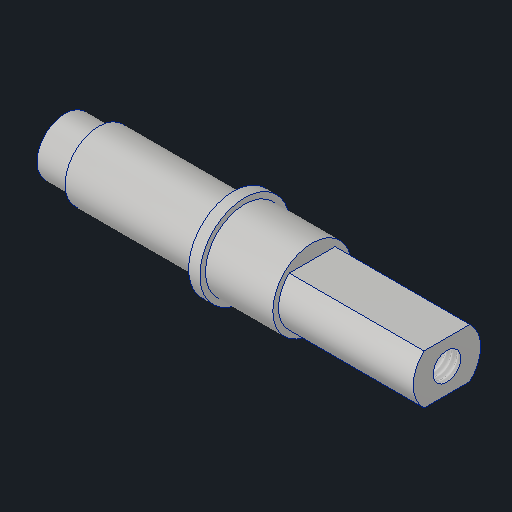
# Autodesk Inventor part: Wał koła
Saved by Autodesk Inventor 2023 (Build 270158000, 158)
## iProperties
Created: 2020-02-09
Part Number: Wał koła
Material: Aluminum 6061
Document SubType Name: Modeling
Designer: SKYNET
Density: 2.7 g/cm^3
Appearance: Aluminum - Flat
Mass: 2.47378 g
Surface Area: 8.25416 cm^2
Volume: 0.916215 cm^3
Author: SKYNET
Autodesk Inventor part; units mm, degrees
ref_plane "YZ Plane" through (0, 0, 0) normal (1, 0, 0) x (0, 1, 0)
ref_plane "XZ Plane" through (0, 0, 0) normal (0, 1, 0) x (-1, 0, 0)
ref_plane "XY Plane" through (0, 0, 0) normal (0, 0, 1) x (1, 0, 0)
sketch "Sketch1" plane through (0, 0, 0) normal (0, 0, 1) x (1, 0, 0)
  line L0 (4, 3) -> (6, 3)
  line L1 (6, 3) -> (6, 3)
  line L2 (16.5, 3.5) -> (16.5, 3.5)
  line L3 (35, 3) -> (35, 0)
  line L4 (4, 3) -> (4, 2.5)
  line L5 (4, 2.5) -> (1, 2.5)
  line L6 (1, 2.5) -> (1, 0)
  line L7 (1, 0) -> (35, 0)
  line L8 (23, 3) -> (35, 3)
  line L9 (23, 3.5) -> (17, 3.5)
  line L10 (23, 3.5) -> (23, 3)
  line L11 (17, 3.5) -> (17, 4)
  line L12 (17, 4) -> (16, 4)
  line L13 (16, 4) -> (16, 3)
  line L14 (6, 3) -> (16, 3)
  point P0 (0, 0)
  dimension "d1" = 2
  dimension "d25" = 3
  dimension "d26" = 2.5
  dimension "d40" = 12
  dimension "d41" = 3
  dimension "d42" = 0.5
  dimension "d44" = 6
  dimension "d45" = 1
  dimension "d46" = 10
  dimension "d47" = 3
  dimension "d48" = 3
  constraints: 30 end point, 6 horizontal, 6 vertical, 4 perpendicular
  measures "d1" distance of L0.start L0.end
  measures "d25" distance of L4.end L5.end
  measures "d26" distance of L5.end L6.end
  measures "d40" distance of L8.start L3.start
  measures "d41" distance of L3.start L3.end
  measures "d42" distance of L9.end L11.end
  measures "d44" distance of L9.start L9.end
  measures "d45" distance of L11.end L12.end
  measures "d46" distance of L1.end L13.end
  measures "d47" distance between parallel lines of L7 L14
  measures "d48" distance between parallel lines of L7 L0
revolve "Revolution2" add sketch "Sketch1" angle 360 about axis through (1, 0, 0) along (1, 0, 0)
sketch "Sketch3" plane through (35, 0, 0) normal (1, 0, 0) x (0, 0, -1)
  circle A0 centre (0, 0) radius 3 projected
  line L0 (-1.6583, 2.5) -> (1.6583, 2.5)
  line L1 (-1.6583, -2.5) -> (1.6583, -2.5)
  point P0 (0, 0)
  dimension "d21" = 0.5
  dimension "d31" = 0.5
  constraints: 4 end point, 4 point on circle, 2 horizontal
  measures "d21" distance edge to line of A0 L0
  measures "d31" distance edge to line of A0 L1
extrude "Extrusion2" [suppressed]
sketch "Sketch4" plane through (4, 0, 0) normal (-1, 0, 0) x (0, 0, 1)
  line L0 (-1.6583, 2.5) -> (1.6583, 2.5)
  circle A0 centre (0, 0) radius 3 projected
  line L1 (-1.6583, -2.5) -> (1.6583, -2.5)
  point P0 (0, 0)
  dimension "d27" = 0.5
  dimension "d30" = 0.5
  constraints: 4 end point, 4 point on circle, 2 horizontal
  measures "d27" distance edge to line of A0 L0
  measures "d30" distance edge to line of A0 L1
extrude "Extrusion3" [suppressed]
sketch "Sketch5" plane through (35, 0, 0) normal (1, 0, 0) x (0, 0, -1)
  point P0 (0, 0)
  point P1 (0, 0)
  constraints: 1 coincident
hole "Hole1" at (35, 0, 0) direction (-1, 0, 0) diameter 2.459 depth 10 tip angle 118 thread size "M3x0.5" class "6H" standard "ISO Metric profile"
sketch "Sketch6" plane through (35, 0, 0) normal (1, 0, 0) x (0, 0, -1)
  circle A0 centre (0, 0) radius 1.2295 projected
  circle A1 centre (0, 0) radius 3 projected
  circle A2 centre (0, 0) radius 3 projected
  line L0 (-2.0396, 2.2) -> (2.0396, 2.2)
  line L1 (-2.0396, -2.2) -> (2.0396, -2.2)
  dimension "d56" = 2.2
  dimension "d57" = 2.2
  constraints: 4 end point, 4 point on circle, 1 horizontal, 1 parallel
  measures "d56" distance from line of point (0, 0) L0
  measures "d57" distance from line of point (0, 0) L1
extrude "Extrusion4" cut sketch "Sketch6" against normal up to surface (12 mm away) contours L0 A1 | A1 L1
equation "\"d57\" = d56"
body "Solid2"
